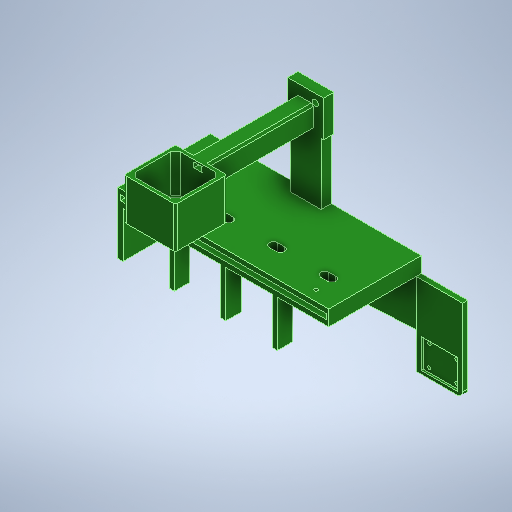
# Autodesk Inventor part: Base
Saved by Autodesk Inventor 2025.4 (Build 294407000, 407)
## iProperties
Created: 2026-03-12
Part Number: Base
Material: Generic
Document SubType Name: Modeling
Designer: lenovo
Density: 1 g/cm^3
Appearance: Default(1)
Author: lenovo
Autodesk Inventor part; units mm, degrees
ref_plane "YZ Plane" through (0, 0, 0) normal (1, 0, 0) x (0, 1, 0)
ref_plane "XZ Plane" through (0, 0, 0) normal (0, 1, 0) x (-1, 0, 0)
ref_plane "XY Plane" through (0, 0, 0) normal (0, 0, 1) x (1, 0, 0)
sketch "Sketch1" plane through (0, 0, 0) normal (0, 0, 1) x (1, 0, 0)
  line L0 (-102.5, -30) -> (102.5, -30)
  line L1 (102.5, -30) -> (102.5, 30)
  line L2 (102.5, 30) -> (-102.5, 30)
  line L3 (-102.5, 30) -> (-102.5, -30)
  line L4 (-102.5, -30) -> (102.5, 30) construction
  line L5 (102.5, -30) -> (-102.5, 30) construction
  point P0 (0, 0)
  dimension "d0" = 205
  dimension "d1" = 60
  constraints: 12 end point, 2 midpoint, 2 parallel, 1 horizontal, 1 perpendicular
  measures "d0" distance of L2.end L1.end
  measures "d1" distance between parallel lines of L0 L2
extrude "Extrusion1" add sketch "Sketch1" along normal blind 90
sketch "Sketch2" plane through (0, 0, 90) normal (0, 0, 1) x (1, 0, 0)
  line L0 (-100.1, 25) -> (100.1, 25)
  line L1 (100.1, 25) -> (100.1, 19.9)
  line L2 (100.1, 19.9) -> (-100.1, 19.9)
  line L3 (-100.1, 19.9) -> (-100.1, 25)
  line L4 (-100.1, 25) -> (100.1, 19.9) construction
  line L5 (100.1, 25) -> (-100.1, 19.9) construction
  line L6 (102.5, 30) -> (-102.5, 30) projected
  point P0 (0, 0)
  point P1 (0, 22.45)
  dimension "d4" = 200.2
  dimension "d5" = 5.1
  dimension "d6" = 5
  constraints: 12 end point, 2 midpoint, 2 parallel, 1 horizontal, 1 perpendicular, 1 vertical alignment
  measures "d4" distance of L1.end L2.end
  measures "d5" distance between parallel lines of L0 L2
  measures "d6" distance between parallel lines of L6 L0
extrude "Extrusion2" cut sketch "Sketch2" against normal blind 20
sketch "Sketch3" plane through (0, 0, 90) normal (0, 0, 1) x (1, 0, 0)
  line L0 (-97.5, -30) -> (102.5, -30)
  line L1 (102.5, -30) -> (102.5, 14.9)
  line L2 (102.5, 14.9) -> (-97.5, 14.9)
  line L3 (-97.5, 14.9) -> (-97.5, -30)
  line L4 (100.1, 19.9) -> (-100.1, 19.9) projected
  line L5 (-102.5, 30) -> (-102.5, -30) projected
  line L6 (102.5, -30) -> (102.5, 30) projected
  line L7 (-102.5, -30) -> (102.5, -30) projected
  point P0 (0, 0)
  point P1 (2.5, -30)
  point P2 (102.5, 0)
  dimension "d9" = 5
  dimension "d10" = 5
  constraints: 8 end point, 2 midpoint, 2 parallel, 2 point on line, 1 horizontal, 1 perpendicular
  measures "d9" distance between parallel lines of L4 L2
  measures "d10" distance between parallel lines of L5 L3
extrude "Extrusion3" cut sketch "Sketch3" against normal blind 65
sketch "Sketch4" plane through (-97.5, 14.9, 90) normal (0, -1, 0) x (1, 0, 0)
  line L0 (200, 0) -> (-5, 0) projected
  line L1 (45, 0) -> (50, 0)
  line L2 (50, 0) -> (50, -15)
  line L3 (50, -15) -> (45, -15)
  line L4 (45, -15) -> (45, 0)
  line L5 (0, -65) -> (0, 0) projected
  line L6 (95, 0) -> (100, 0)
  line L7 (100, 0) -> (100, -15)
  line L8 (100, -15) -> (95, -15)
  line L9 (95, -15) -> (95, 0)
  line L10 (145, 0) -> (150, 0)
  line L11 (150, 0) -> (150, -15)
  line L12 (150, -15) -> (145, -15)
  line L13 (145, -15) -> (145, 0)
  point P0 (97.5, -90)
  dimension "d14" = 5
  dimension "d15" = 15
  dimension "d16" = 45
  dimension "d19" = 50
  constraints: 24 end point, 2 horizontal, 2 parallel, 1 perpendicular, 1 point on line, 16 other
  measures "d14" distance between parallel lines of L4 L2
  measures "d15" distance from line of L3 L1.start
  measures "d16" distance between parallel lines of L5 L4
  measures "d19" distance of L1.start L6.start
extrude "Extrusion4" add sketch "Sketch4" along normal up to surface (44.9 mm away)
sketch "Sketch7" plane through (-102.5, -30, 0) normal (0, -1, 0) x (1, 0, 0)
  line L0 (5, 90) -> (5, 25) projected
  arc A0 (5, 25) -> (14.4751, 15.0138) centre (15, 25) ccw
  line L1 (5, 25) -> (205, 25) projected
  line L2 (14.4751, 15.0138) -> (205, 5)
  line L3 (205, 0) -> (205, 25) projected
  line L4 (205, 8) -> (205, 25)
  line L5 (0, 0) -> (205, 0) projected
  point P0 (102.5, 0)
  dimension "d45" = 10
  dimension "d169" = 5
  constraints: 4 end point, 2 point on circle, 2 point on line, 2 tangent, 1 centre point
  measures "d45" distance from line of L0 A0.centre
  measures "d169" distance from line of L5 L2.end
extrude "Extrusion7" cut sketch "Sketch7" against normal up to surface (44.9 mm away)
sketch "Sketch9" plane through (-102.5, 30, 0) normal (0, 1, 0) x (1, 0, 0)
  circle A0 centre (27.5, -63) radius 5.25
  line L0 (5, -90) -> (5, -25) projected
  line L1 (2.4, -70) -> (202.6, -70) projected
  line L2 (31, -63) -> (24, -63) construction
  line L3 (31, -59) -> (24, -59)
  line L4 (24, -67) -> (31, -67)
  arc A1 (31, -67) -> (31, -59) centre (31, -63) ccw
  arc A2 (24, -59) -> (24, -67) centre (24, -63) ccw
  point P0 (102.5, 0)
  point P1 (20, -63)
  point P2 (35, -63)
  dimension "d48" = 10.5
  dimension "d49" = 22.5
  dimension "d50" = 7
  dimension "d187" = 8
  dimension "d188" = 15
  constraints: 8 end point, 6 point on circle, 4 tangent, 3 centre point, 1 horizontal, 1 midpoint, 1 parallel
  measures "d48" diameter of A0
  measures "d49" distance from line of L0 A0.centre
  measures "d50" distance from line of L1 A0.centre
  measures "d187" distance between parallel lines of L4 L3
  measures "d188" distance of point (20, -63) point (35, -63)
extrude "Extrusion8" cut sketch "Sketch9" against normal through all contours A0 L4 L3 | A0 L3 A1 L4 | A0 L4 A2 L3
sketch "Sketch11" plane through (-102.5, 30, 0) normal (0, 1, 0) x (1, 0, 0)
  line L0 (205, 0) -> (0, 0) projected
  line L1 (117.5, 0) -> (87.5, 0)
  line L2 (87.5, 0) -> (87.5, -10)
  line L3 (87.5, -10) -> (117.5, -10)
  line L4 (117.5, -10) -> (117.5, 0)
  point P0 (102.5, 0)
  point P1 (87.5, 0)
  point P2 (102.5, 0)
  point P3 (102.5, 0)
  dimension "d56" = 30
  dimension "d57" = 10
  constraints: 8 end point, 2 midpoint, 2 parallel, 1 coincident, 1 horizontal, 1 perpendicular, 1 point on line
  measures "d56" distance of L3.end L2.end
  measures "d57" distance of L2.end L1.end
extrude "Extrusion10" add sketch "Sketch11" along normal blind 60
sketch "Sketch12" plane through (0, 0, 0) normal (0, 0, -1) x (-1, 0, 0)
  line L0 (-17.5, 125) -> (17.5, 125)
  line L1 (17.5, 125) -> (17.5, 90)
  line L2 (17.5, 90) -> (-17.5, 90)
  line L3 (-17.5, 90) -> (-17.5, 125)
  line L4 (-15, 90) -> (15, 90) projected
  point P0 (0, 0)
  point P1 (-102.5, 65)
  point P2 (0, 90)
  dimension "d60" = 35
  constraints: 8 end point, 2 parallel, 2 perpendicular, 1 horizontal, 1 midpoint, 2 other
  measures "d60" distance of L1.end L2.end
extrude "Extrusion11" add sketch "Sketch12" against normal blind 10
sketch "Sketch13" plane through (-15, 30, 10) normal (0, 0, 1) x (1, 0, 0)
  line L0 (7.5, 85) -> (22.5, 85)
  line L1 (22.5, 85) -> (22.5, 63)
  line L2 (22.5, 63) -> (7.5, 63)
  line L3 (7.5, 63) -> (7.5, 85)
  line L4 (-2.5, 95) -> (-2.5, 60) projected
  line L5 (32.5, 95) -> (-2.5, 95) projected
  line L6 (22.5, 85) -> (7.5, 85)
  point P0 (15, -30)
  point P1 (-2.5, 77.5)
  point P2 (7.5, 74)
  point P3 (15, 95)
  point P4 (15, 85)
  point P5 (-2.5, 77.5)
  point P6 (15, 85)
  point P7 (15, 95)
  dimension "d63" = 15
  dimension "d146" = 22
  dimension "d164" = 10
  constraints: 10 end point, 7 midpoint, 2 horizontal, 2 parallel, 2 vertical alignment, 1 perpendicular
  measures "d63" distance of L0.start L0.end
  measures "d146" distance of L2.end L0.start
  measures "d164" distance between parallel lines of L5 L0
extrude "Extrusion12" add sketch "Sketch13" along normal blind 101.5
sketch "Sketch14" plane through (-15, 30, 111.5) normal (0, 0, 1) x (1, 0, 0)
  line L0 (-10, 85) -> (40, 85)
  line L1 (40, 85) -> (40, 45)
  line L2 (40, 45) -> (-10, 45)
  line L3 (-10, 45) -> (-10, 85)
  line L4 (-10, 85) -> (40, 45) construction
  line L5 (40, 85) -> (-10, 45) construction
  line L6 (22.5, 63) -> (22.5, 85) projected
  line L7 (22.5, 85) -> (7.5, 85) projected
  point P0 (15, -30)
  point P1 (15, 65)
  point P2 (22.5, 74)
  point P3 (15, 85)
  point P4 (15, 85)
  point P5 (15, 85)
  dimension "d67" = 40
  dimension "d68" = 50
  constraints: 12 end point, 7 midpoint, 2 parallel, 1 horizontal, 1 perpendicular, 1 vertical alignment
  measures "d67" distance of L2.end L0.start
  measures "d68" distance of L0.start L0.end
extrude "Extrusion13" add sketch "Sketch14" along normal blind 50
sketch "Sketch15" plane through (-25, 75, 111.5) normal (0, -1, 0) x (1, 0, 0)
  line L0 (3.25, 46.75) -> (46.75, 46.75)
  line L1 (46.75, 46.75) -> (46.75, 3.25)
  line L2 (46.75, 3.25) -> (3.25, 3.25)
  line L3 (3.25, 3.25) -> (3.25, 46.75)
  line L4 (3.25, 46.75) -> (46.75, 3.25) construction
  line L5 (46.75, 46.75) -> (3.25, 3.25) construction
  line L6 (0, 0) -> (0, 50) projected
  line L7 (0, 50) -> (50, 50) projected
  point P0 (25, -111.5)
  point P1 (25, 25)
  point P2 (0, 25)
  point P3 (25, 50)
  dimension "d71" = 43.5
  constraints: 12 end point, 4 midpoint, 2 parallel, 2 perpendicular, 1 horizontal, 1 horizontal alignment, 1 vertical alignment
  measures "d71" distance of L1.end L2.end
extrude "Extrusion14" cut sketch "Sketch15" against normal blind 50
sketch "Sketch16" plane through (-25, 75, 111.5) normal (0, -1, 0) x (1, 0, 0)
  line L0 (3.25, 46.75) -> (46.75, 46.75)
  line L1 (46.75, 46.75) -> (46.75, 3.25)
  line L2 (46.75, 3.25) -> (3.25, 3.25)
  line L3 (3.25, 3.25) -> (3.25, 46.75)
  line L4 (3.25, 46.75) -> (46.75, 3.25) construction
  line L5 (46.75, 46.75) -> (3.25, 3.25) construction
  line L6 (0, 0) -> (0, 50) projected
  line L7 (0, 50) -> (50, 50) projected
  circle A0 centre (8.25, 41.75) radius 1.65
  circle A1 centre (41.75, 41.75) radius 1.65
  circle A2 centre (41.75, 41.75) radius 1.65
  circle A3 centre (8.25, 8.25) radius 1.65
  circle A4 centre (41.75, 8.25) radius 1.65
  circle A5 centre (25, 25) radius 11
  point P0 (25, -111.5)
  point P1 (0, 25)
  point P2 (25, 50)
  dimension "d74" = 43.5
  dimension "d75" = 3.3
  dimension "d76" = 5
  dimension "d77" = 3.3
  dimension "d78" = 5
  dimension "d81" = 33.5
  dimension "d84" = 33.5
  dimension "d87" = 22
  constraints: 12 end point, 6 centre point, 4 midpoint, 2 horizontal, 2 parallel, 2 perpendicular, 2 point on line, 1 coincident, 1 horizontal alignment, 1 vertical, 1 vertical alignment, 6 other
  measures "d74" distance of L1.end L2.end
  measures "d75" diameter of A0
  measures "d76" distance from line of L0 A0.centre
  measures "d77" diameter of A1
  measures "d78" distance from line of L0 A1.centre
  measures "d81" distance of A0.centre A2.centre
  measures "d84" distance of A0.centre A3.centre
  measures "d87" diameter of A5
extrude "Extrusion15" add sketch "Sketch16" against normal blind 3
chamfer "Chamfer1" distance 4.5 angle 45 4 edges at (-21.75, 96.5, 114.75) (-21.75, 96.5, 158.25) (21.75, 96.5, 114.75) (21.75, 96.5, 158.25)
fillet "Fillet2" radius 2 4 edges at (25, 95, 161.5) (-25, 95, 161.5) (25, 95, 111.5) (-25, 95, 111.5)
sketch "Sketch17" plane through (0, 0, 0) normal (0, 0, 1) x (1, 0, 0)
  circle A0 centre (-92.5, -20) radius 1.65
  line L0 (-102.5, 30) -> (-102.5, -30) projected
  line L1 (-83.3079, -30) -> (-97.5, -30) projected
  circle A1 centre (9.5, 117) radius 1.65
  line L2 (17.5, 125) -> (-17.5, 125) projected
  line L3 (17.5, 90) -> (17.5, 125) projected
  line L4 (-102.5, -30) -> (102.5, -30) projected
  point P0 (0, 0)
  dimension "d94" = 3.3
  dimension "d95" = 10
  dimension "d97" = 3.3
  dimension "d98" = 8
  dimension "d99" = 8
  dimension "d170" = 10
  constraints: 2 centre point
  measures "d94" diameter of A0
  measures "d95" distance from line of L0 A0.centre
  measures "d97" diameter of A1
  measures "d98" distance from line of L2 A1.centre
  measures "d99" distance from line of L3 A1.centre
  measures "d170" distance from line of L4 A0.centre
extrude "Extrusion16" cut sketch "Sketch17" along normal blind 5
sketch "Sketch20" plane through (0, 0, 0) normal (0, 0, -1) x (-1, 0, 0)
  circle A0 centre (92.5, -20) radius 1.65 projected
  circle A1 centre (92.5, -20) radius 3
  circle A2 centre (-9.5, 117) radius 3
  circle A3 centre (-9.5, 117) radius 1.65 projected
  point P0 (0, 0)
  dimension "d106" = 6
  dimension "d107" = 6
  constraints: 2 centre point, 1 coincident, 1 concentric
  measures "d106" diameter of A1
  measures "d107" diameter of A2
extrude "Extrusion18" cut sketch "Sketch20" against normal blind 50 from surface at -5 contours A0 | A1 | A2 | A3
sketch "Sketch23" plane through (-102.5, -30, 0) normal (0, -1, 0) x (1, 0, 0)
  line L0 (206.0756, 24.942) -> (19.1921, 35.0218) projected
  line L1 (205, 5) -> (250, 5)
  line L2 (250, 5) -> (250, 0)
  line L3 (250, 0) -> (205, 0)
  line L4 (205, 0) -> (205, 5)
  point P0 (102.5, 0)
  dimension "d111" = 45
  constraints: 8 end point, 2 parallel, 1 coincident, 1 horizontal, 1 perpendicular
  measures "d111" distance of L2.end L3.end
extrude "Extrusion19" add sketch "Sketch23" along normal blind 35
extrude "Extrusion20" add sketch "Sketch23" against normal up to surface (44.9 mm away)
sketch "Sketch24" plane through (102.5, -65, 5) normal (0, 0, 1) x (1, 0, 0)
  circle A0 centre (37.25, 7.25) radius 1.65
  line L0 (45, 79.9) -> (45, 0) projected
  line L1 (45, 0) -> (0, 0) projected
  line L2 (5.75, 30.75) -> (39.25, 30.75)
  line L3 (39.25, 30.75) -> (39.25, 4.25)
  line L4 (39.25, 4.25) -> (5.75, 4.25)
  line L5 (5.75, 4.25) -> (5.75, 30.75)
  line L6 (0, 35) -> (0, 0) projected
  line L7 (5.75, 17.5) -> (39.25, 17.5)
  circle A1 centre (37.25, 27.75) radius 1.65
  circle A2 centre (10.75, 27.75) radius 1.65
  circle A3 centre (10.75, 7.25) radius 1.65
  line L8 (4.75, 31.75) -> (40.25, 31.75)
  line L9 (40.25, 31.75) -> (40.25, 3.25)
  line L10 (40.25, 3.25) -> (4.75, 3.25)
  line L11 (4.75, 3.25) -> (4.75, 31.75)
  point P0 (-102.5, 65)
  point P1 (45, 34.9)
  point P2 (0, 17.5)
  point P3 (22.5, 30.75)
  point P4 (22.5, 0)
  dimension "d118" = 3.3
  dimension "d120" = 33.5
  dimension "d121" = 26.5
  dimension "d123" = 3
  dimension "d124" = 2
  dimension "d125" = 3.3
  dimension "d126" = 3
  dimension "d127" = 5
  dimension "d142" = 1
  constraints: 18 end point, 5 midpoint, 4 centre point, 4 parallel, 2 perpendicular, 2 symmetric about line, 1 horizontal, 1 horizontal alignment, 1 vertical alignment, 5 other
  measures "d118" diameter of A0
  measures "d120" distance of L2.start L2.end
  measures "d121" distance of L2.end L3.end
  measures "d123" distance from line of L4 A0.centre
  measures "d124" distance from line of L3 A0.centre
  measures "d125" diameter of A2
  measures "d126" distance from line of L2 A2.centre
  measures "d127" distance from line of L5 A2.centre
  measures "d142" distance between parallel lines of L5 L11
extrude "Extrusion21" cut sketch "Sketch24" against normal blind 10 contours A0 | A1 | A2 | A3
extrude "Extrusion24" cut sketch "Sketch24" against normal blind 2 contours L2 L3 L7 L5 | L7 L3 L4 L5 | L8 L9 L10 L11
fillet "Fillet4" radius 5 1 edges at (147.5, -65, 2.5)
sketch "Sketch27" plane through (-17.25, 115, 114.75) normal (0, 0, 1) x (1, 0, 0)
  line L0 (13.25, -2) -> (21.25, -2)
  line L1 (21.25, -2) -> (21.25, -7)
  line L2 (21.25, -7) -> (13.25, -7)
  line L3 (13.25, -7) -> (13.25, -2)
  line L4 (0, 0) -> (34.5, 0) projected
  point P0 (17.25, -115)
  point P1 (17.25, -2)
  point P2 (17.25, 0)
  dimension "d150" = 8
  dimension "d151" = 5
  dimension "d154" = 2
  constraints: 8 end point, 2 midpoint, 2 parallel, 1 horizontal, 1 perpendicular, 1 vertical alignment
  measures "d150" distance of L1.end L2.end
  measures "d151" distance of L0.end L1.end
  measures "d154" distance between parallel lines of L4 L0
extrude "Extrusion25" cut sketch "Sketch27" against normal through all
ref_plane "Work Plane1" through (0, 93, 10) normal (1, 0, 0) x (0, 0, -1)
pattern_linear "Rectangular Pattern1" count 4 spacing 50 along (1, 0, 0) of "Extrusion8"
sketch "Sketch29" plane through (-7.5, 93, 10) normal (-1, 0, 0) x (0, 0, 1)
  line L0 (104.75, 20) -> (-10, 20) projected
  line L1 (104.75, 15) -> (-10, 15) projected
  line L2 (25, 20) -> (10, 20)
  line L3 (10, 20) -> (10, 15)
  line L4 (10, 15) -> (25, 15)
  line L5 (25, 15) -> (25, 20)
  line L6 (0, 32) -> (0, -3) projected
  point P0 (-10, -93)
  point P1 (10, 20)
  dimension "d171" = 10
  dimension "d172" = 15
  constraints: 8 end point, 2 parallel, 2 point on line, 1 horizontal, 1 perpendicular
  measures "d171" distance between parallel lines of L6 L3
  measures "d172" distance between parallel lines of L3 L5
extrude "Extrusion26" cut sketch "Sketch29" against normal up to next contours L5 L1 L3 L0
sketch "Sketch30" plane through (52.5, 14.9, 90) normal (0, -1, 0) x (1, 0, 0)
  circle A0 centre (27.6, -10) radius 1.65
  circle A1 centre (-132.6, -10) radius 1.65
  line L0 (47.6, -20) -> (-152.6, -20) projected
  line L1 (47.6, 0) -> (47.6, -20) projected
  line L2 (-152.6, 0) -> (-152.6, -20) projected
  point P0 (-52.5, -90)
  dimension "d175" = 3.3
  dimension "d176" = 3.3
  dimension "d177" = 10
  dimension "d178" = 20
  dimension "d179" = 20
  constraints: 2 centre point, 1 horizontal alignment
  measures "d175" diameter of A0
  measures "d176" diameter of A1
  measures "d177" distance from line of L0 A0.centre
  measures "d178" distance from line of L1 A0.centre
  measures "d179" distance from line of L2 A1.centre
extrude "Extrusion27" cut sketch "Sketch30" against normal blind 94.5
sketch "Sketch31" plane through (52.5, 14.9, 90) normal (0, -1, 0) x (1, 0, 0)
  circle A0 centre (-132.6, -10) radius 1.65 projected
  circle A1 centre (-132.6, -10) radius 3
  circle A2 centre (27.6, -10) radius 1.65 projected
  circle A3 centre (27.6, -10) radius 3
  point P0 (-52.5, -90)
  dimension "d182" = 6
  dimension "d183" = 6
  constraints: 2 centre point, 2 coincident, 1 horizontal alignment
  measures "d182" diameter of A1
  measures "d183" diameter of A3
extrude "Extrusion28" cut sketch "Sketch31" against normal blind 2
chamfer "Chamfer2" distance 2 angle 45 3 edges at (-7.5, 93, 60.75) (7.5, 115, 83.25) (7.5, 93, 60.75)
body "Solid1"
